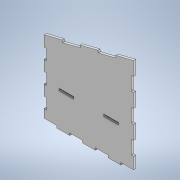
# Autodesk Inventor part: back
Saved by Autodesk Inventor 2020 (Build 240168000, 168)
## iProperties
Created: 2020-02-22
Part Number: back
Material: Generic
Document SubType Name: Modeling
Designer: udvarhelyi
Density: 1 g/cm^3
Appearance: Default
Author: udvarhelyi
Autodesk Inventor part; units mm, degrees
ref_plane "YZ Plane" through (0, 0, 0) normal (1, 0, 0) x (0, 1, 0)
ref_plane "XZ Plane" through (0, 0, 0) normal (0, 1, 0) x (-1, 0, 0)
ref_plane "XY Plane" through (0, 0, 0) normal (0, 0, 1) x (1, 0, 0)
sketch "Sketch1" plane through (0, 0, 0) normal (0, 0, 1) x (1, 0, 0)
  line L0 (0, 85.7143) -> (3, 85.7143)
  line L1 (3, 71.4286) -> (0, 71.4286)
  line L2 (0, 57.1429) -> (3, 57.1429)
  line L3 (3, 42.8571) -> (0, 42.8571)
  line L4 (0, 28.5714) -> (3, 28.5714)
  line L5 (3, 14.2857) -> (0, 14.2857)
  line L6 (117, 18.5714) -> (120, 18.5714)
  line L7 (120, 37.1429) -> (117, 37.1429)
  line L8 (117, 55.7143) -> (120, 55.7143)
  line L9 (120, 74.2857) -> (117, 74.2857)
  line L10 (117, 92.8571) -> (120, 92.8571)
  line L11 (120, 111.4286) -> (117, 111.4286)
  line L12 (17.1429, 3) -> (17.1429, 0)
  line L13 (34.2857, 0) -> (34.2857, 3)
  line L14 (51.4286, 3) -> (51.4286, 0)
  line L15 (68.5714, 0) -> (68.5714, 3)
  line L16 (85.7143, 3) -> (85.7143, 0)
  line L17 (102.8571, 0) -> (102.8571, 3)
  line L18 (2.344, 3) -> (0, 3)
  line L19 (102.8571, 3) -> (120, 3)
  line L20 (17.1429, 3) -> (2.344, 3)
  line L21 (51.4286, 3) -> (34.2857, 3)
  line L22 (85.7143, 3) -> (68.5714, 3)
  line L23 (17.1429, 0) -> (34.2857, 0)
  line L24 (51.4286, 0) -> (68.5714, 0)
  line L25 (85.7143, 0) -> (102.8571, 0)
  line L26 (117, 37.1429) -> (117, 18.5714)
  line L27 (117, 111.4286) -> (117, 92.8571)
  line L28 (117, 74.2857) -> (117, 55.7143)
  line L29 (120, 111.4286) -> (120, 130)
  line L30 (120, 74.2857) -> (120, 92.8571)
  line L31 (120, 3) -> (120, 18.5714)
  line L32 (120, 37.1429) -> (120, 55.7143)
  line L33 (3, 71.4286) -> (3, 85.7143)
  line L34 (3, 14.2857) -> (3, 28.5714)
  line L35 (3, 42.8571) -> (3, 57.1429)
  line L36 (0, 14.2857) -> (0, 3)
  line L37 (0, 42.8571) -> (0, 28.5714)
  line L38 (0, 100) -> (0, 85.7143)
  line L39 (0, 71.4286) -> (0, 57.1429)
  line L40 (24, 106) -> (24.7276, 103.0896)
  line L41 (48, 112) -> (48.7276, 109.0896)
  line L42 (72, 118) -> (72.7276, 115.0896)
  line L43 (96, 124) -> (96.7276, 121.0896)
  line L44 (24, 106) -> (0, 100)
  line L45 (120, 130) -> (96, 124)
  line L46 (72, 118) -> (48, 112)
  line L47 (24.7276, 103.0896) -> (48.7276, 109.0896)
  line L48 (72.7276, 115.0896) -> (96.7276, 121.0896)
  point P0 (0, 0)
  point P1 (0, 0)
  dimension "d32" = 100
  dimension "d33" = 3
  dimension "d34" = 130
  dimension "d35" = 17.1429
  dimension "d36" = 34.2857
  dimension "d37" = 51.4286
  dimension "d38" = 85.7143
  dimension "d39" = 68.5714
  dimension "d40" = 102.8571
  dimension "d41" = 120
  dimension "d42" = 3
  dimension "d43" = 18.5714
  dimension "d44" = 55.7143
  dimension "d45" = 111.4286
  dimension "d46" = 92.8571
  dimension "d47" = 37.1429
  dimension "d48" = 74.2857
  dimension "d49" = 14.2857
  dimension "d50" = 28.5714
  dimension "d51" = 42.8571
  dimension "d52" = 57.1429
  dimension "d53" = 71.4286
  dimension "d54" = 85.7143
  dimension "d55" = 3
  dimension "d56" = 3
  dimension "d58" = 24.7386
  dimension "d59" = 49.4773
  dimension "d60" = 74.2159
  dimension "d61" = 98.9545
  dimension "d62" = 3
  dimension "d71" = 3
  constraints: 98 end point, 73 perpendicular, 29 parallel, 19 collinear, 4 vertical, 1 coincident, 1 point on line, 1 other
  measures "d32" distance of L38.start point (0, 0)
  measures "d33" distance from line of point (0, 0) L21
  measures "d34" vertical distance of point (0, 0) L29.end
  measures "d35" distance from line of point (0, 0) L12
  measures "d36" distance from line of point (0, 0) L13
  measures "d37" distance from line of point (0, 0) L14
  measures "d38" distance from line of point (0, 0) L16
  measures "d39" distance from line of point (0, 0) L15
  measures "d40" distance from line of point (0, 0) L17
  measures "d41" distance from line of point (0, 0) L31
  measures "d42" distance of L6.start L6.end
  measures "d43" distance from line of point (0, 0) L6
  measures "d44" distance from line of point (0, 0) L8
  measures "d45" vertical distance of point (0, 0) L11.start
  measures "d46" vertical distance of point (0, 0) L10.end
  measures "d47" vertical distance of point (0, 0) L7.end
  measures "d48" distance from line of point (0, 0) L9
  measures "d49" distance of L5.end point (0, 0)
  measures "d50" vertical distance of point (0, 0) L4.end
  measures "d51" vertical distance of point (0, 0) L3.start
  measures "d52" distance of point (0, 0) L2.start
  measures "d53" distance of point (0, 0) L1.end
  measures "d54" distance of point (0, 0) L0.start
  measures "d55" distance of L5.start L5.end
  measures "d56" distance from line of point (0, 0) L34
  measures "d58" distance from line of L38.start L40
  measures "d59" distance from line of L38.start L41
  measures "d60" distance from line of L38.start L42
  measures "d61" distance from line of L38.start L43
  measures "d62" distance between parallel lines of L48 L46
  measures "d71" distance of L13.start L13.end
extrude "Extrusion1" add sketch "Sketch1" along normal blind 3
sketch "Sketch2" plane through (0, 0, 3) normal (0, 0, 1) x (1, 0, 0)
  line L0 (20, 45) -> (40, 45)
  line L1 (40, 45) -> (40, 48)
  line L2 (40, 48) -> (20, 48)
  line L3 (20, 48) -> (20, 45)
  line L4 (17.1429, 0) -> (34.2857, 0) projected
  line L5 (0, 42.8571) -> (0, 28.5714) projected
  line L6 (80, 45) -> (100, 45)
  line L7 (100, 45) -> (100, 48)
  line L8 (100, 48) -> (80, 48)
  line L9 (80, 48) -> (80, 45)
  line L10 (120, 37.1429) -> (120, 55.7143) projected
  point P0 (0, 0)
  dimension "d63" = 3
  dimension "d64" = 45
  dimension "d65" = 20
  dimension "d66" = 20
  dimension "d67" = 20
  dimension "d68" = 20
  constraints: 16 end point, 4 parallel, 2 collinear, 2 horizontal, 2 perpendicular
  measures "d63" distance of L2.end L0.start
  measures "d64" distance between parallel lines of L4 L0
  measures "d65" distance of L1.end L2.end
  measures "d66" distance between parallel lines of L5 L3
  measures "d67" distance of L7.end L8.end
  measures "d68" distance between parallel lines of L10 L7
extrude "Extrusion2" cut sketch "Sketch2" against normal through all
equation "\"d32\" = height_front"
equation "\"d33\" = tt"
equation "\"d34\" = height_back"
equation "\"d35\" = 0.142857 * ht - tol"
equation "\"d36\" = 0.285714 * ht + tol"
equation "\"d37\" = 0.428571 * ht - tol"
equation "\"d38\" = 0.714286 * ht - tol"
equation "\"d39\" = 0.571429 * ht + tol"
equation "\"d40\" = 0.857143 * ht + tol"
equation "\"d41\" = ht"
equation "\"d42\" = tt"
equation "\"d43\" = 0.142857 * height_back + tol"
equation "\"d44\" = 0.428571 * height_back + tol"
equation "\"d45\" = 0.857143 * height_back - tol"
equation "\"d46\" = 0.714286 * height_back + tol"
equation "\"d47\" = 0.285714 * height_back - tol"
equation "\"d48\" = 0.571429 * height_back - tol"
equation "\"d49\" = 0.142857 * height_front - tol"
equation "\"d50\" = 0.285714 * height_front + tol"
equation "\"d51\" = 0.428571 * height_front - tol"
equation "\"d52\" = 0.571429 * height_front + tol"
equation "\"d53\" = 0.714286 * height_front - tol"
equation "\"d54\" = 0.857143 * height_front + tol"
equation "\"d55\" = tt"
equation "\"d24\" = tt"
equation "\"ht\" = 120"
equation "\"tt\" = 3"
equation "\"tol\" = 0"
equation "\"height_back\" = 130"
equation "\"height_front\" = 100"
equation "\"d4\" = tt"
equation "\"d31\" = tt"
equation "\"tiroir\" = 1"
equation "\"ht_diag\" = 123.69317"
equation "\"nHoles\" = 4"
equation "\"shelfH\" = 35"
body "Solid1"
